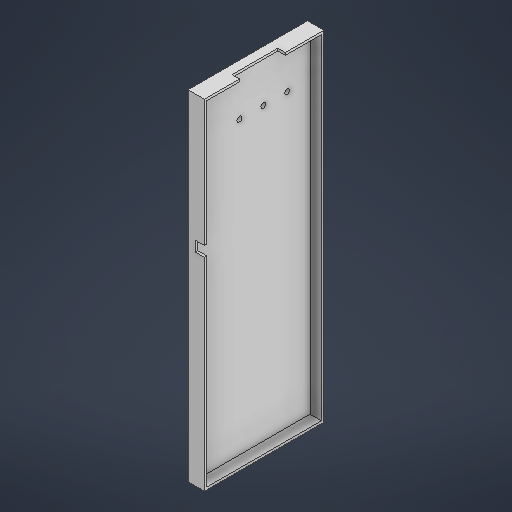
# Autodesk Inventor part: cDAQ_Lid_Box
Saved by Autodesk Inventor 2027 (Build 310192000, 192)
## iProperties
Created: 2026-05-08
Part Number: cDAQ_Lid_Box
Material: Generic
Document SubType Name: Modeling
Designer: giese
Density: 1 g/cm^3
Appearance: Default
Author: giese
Autodesk Inventor part; units mm, degrees
ref_plane "YZ Plane" through (0, 0, 0) normal (1, 0, 0) x (0, 1, 0)
ref_plane "XZ Plane" through (0, 0, 0) normal (0, 1, 0) x (-1, 0, 0)
ref_plane "XY Plane" through (0, 0, 0) normal (0, 0, 1) x (1, 0, 0)
sketch "Sketch1" plane through (0, 0, 0) normal (1, 0, 0) x (0, 1, 0)
  line L0 (50.7569, 48.4212) -> (-212.6919, 48.4212)
  line L1 (-212.6919, 48.4212) -> (-212.6919, -44.2888)
  line L2 (-212.6919, -44.2888) -> (50.7569, -44.2888)
  line L3 (50.7569, -44.2888) -> (50.7569, 48.4212)
  point P0 (0, 0)
  dimension "d0" = 92.71
  dimension "d1" = 263.4488
  constraints: 8 end point, 2 parallel, 1 horizontal, 1 perpendicular
  measures "d0" distance of L2.end L0.start
  measures "d1" distance of L0.start L0.end
extrude "Extrusion1" add sketch "Sketch1" along normal blind 12.7
sketch "Sketch2" plane through (12.7, 0, 0) normal (1, 0, 0) x (0, 0, -1)
  line L0 (-46.5162, 48.8519) -> (42.3838, 48.8519)
  line L1 (42.3838, 48.8519) -> (42.3838, -210.7869)
  line L2 (42.3838, -210.7869) -> (-46.5162, -210.7869)
  line L3 (-46.5162, -210.7869) -> (-46.5162, 48.8519)
  line L4 (-48.4212, 50.7569) -> (-48.4212, -212.6919) projected
  line L5 (-48.4212, -212.6919) -> (44.2888, -212.6919) projected
  point P0 (0, 0)
  dimension "d4" = 88.9
  dimension "d5" = 259.6388
  dimension "d6" = 1.905
  dimension "d7" = 1.905
  constraints: 8 end point, 2 parallel, 1 horizontal, 1 perpendicular
  measures "d4" distance of L0.start L0.end
  measures "d5" distance of L0.end L1.end
  measures "d6" distance between parallel lines of L4 L3
  measures "d7" distance between parallel lines of L5 L2
extrude "Extrusion2" cut sketch "Sketch2" against normal blind 8.89
sketch "Sketch3" plane through (0, 0, 0) normal (-1, 0, 0) x (0, 0, 1)
  circle A0 centre (-24.7054, 14.9125) radius 2
  line L0 (-44.2888, -212.6919) -> (-44.2888, 50.7569) projected
  line L1 (-44.2888, 50.7569) -> (48.4212, 50.7569) projected
  circle A1 centre (-6.2066, 14.9125) radius 2
  circle A2 centre (12.2923, 14.9125) radius 2
  point P0 (0, 0)
  dimension "d10" = 19.5834
  dimension "d11" = 35.8445
  dimension "d12" = 35.8445
  dimension "d13" = 18.4988
  dimension "d14" = 4
  dimension "d15" = 4
  dimension "d16" = 35.8445
  dimension "d17" = 18.4988
  dimension "d18" = 36.9976
  dimension "d21" = 4
  constraints: 3 centre point
  measures "d10" distance from line of L0 A0.centre
  measures "d11" distance from line of L1 A0.centre
  measures "d12" distance from line of L1 A1.centre
  measures "d13" distance of A0.centre A1.centre
  measures "d14" diameter of A1
  measures "d15" diameter of A2
  measures "d16" distance from line of L1 A2.centre
  measures "d17" distance of A1.centre A2.centre
  measures "d18" distance of A0.centre A2.centre
  measures "d21" diameter of A0
extrude "Extrusion3" cut sketch "Sketch3" against normal blind 3.81
sketch "Sketch5" plane through (0, -212.6919, 48.4212) normal (0, 0, 1) x (1, 0, 0)
  line L0 (5.5575, 157.1483) -> (12.7, 157.1483)
  line L1 (12.7, 157.1483) -> (12.7, 165.1483)
  line L2 (12.7, 165.1483) -> (5.5575, 165.1483)
  line L3 (5.5575, 165.1483) -> (5.5575, 157.1483)
  line L4 (12.7, 263.4488) -> (12.7, 0) projected
  line L5 (0, 263.4488) -> (12.7, 263.4488) projected
  point P0 (0, 212.6919)
  point P1 (9.1288, 165.1483)
  point P2 (9.1288, 157.1483)
  dimension "d22" = 8
  dimension "d23" = 7.1425
  dimension "d24" = 0
  dimension "d25" = 98.3005
  constraints: 8 end point, 2 midpoint, 2 parallel, 1 horizontal, 1 perpendicular
  measures "d22" distance of point (9.129, 165.148) point (9.129, 157.148)
  measures "d23" distance between parallel lines of L1 L3
  measures "d24" distance between parallel lines of L4 L1
  measures "d25" distance between parallel lines of L5 L2
extrude "Extrusion4" cut sketch "Sketch5" against normal blind 16.51
sketch "Sketch6" plane through (0, 50.7569, 48.4212) normal (0, 1, 0) x (1, 0, 0)
  line L0 (12.7, 1.905) -> (12.7, 90.805) projected
  line L1 (6.8834, 27.2187) -> (12.7, 27.2187)
  line L2 (12.7, 27.2187) -> (12.7, 62.7888)
  line L3 (12.7, 62.7888) -> (6.8834, 62.7888)
  line L4 (6.8834, 62.7888) -> (6.8834, 27.2187)
  line L5 (0, 92.71) -> (12.7, 92.71) projected
  point P0 (0, 48.4212)
  point P1 (9.7917, 62.7888)
  point P2 (9.7917, 27.2187)
  dimension "d30" = 5.8166
  dimension "d31" = 35.5701
  dimension "d32" = 29.9212
  constraints: 8 end point, 2 midpoint, 2 parallel, 1 horizontal, 1 perpendicular, 1 point on line
  measures "d30" distance between parallel lines of L0 L4
  measures "d31" distance of point (9.792, 62.789) point (9.792, 27.219)
  measures "d32" distance between parallel lines of L5 L3
extrude "Extrusion5" cut sketch "Sketch6" against normal blind 3.81
body "Solid1"
